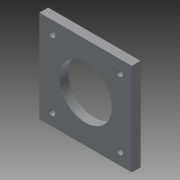
# Autodesk Inventor part: ZMotorMount
Saved by Autodesk Inventor 2015 (Build 190159000, 159)
## iProperties
Created: 2014-08-12
Part Number: ZMotorMount
Material: Generic
Document SubType Name: Modeling
Designer: Jack
Density: 1 g/cm^3
Appearance: Default
Author: Jack
Autodesk Inventor part; units mm, degrees
ref_plane "YZ Plane" through (0, 0, 0) normal (1, 0, 0) x (0, 1, 0)
ref_plane "XZ Plane" through (0, 0, 0) normal (0, 1, 0) x (-1, 0, 0)
ref_plane "XY Plane" through (0, 0, 0) normal (0, 0, 1) x (1, 0, 0)
sketch "Sketch1" plane through (0, 0, 0) normal (0, 1, 0) x (-1, 0, 0)
  line L0 (0, 0) -> (42.3, 0)
  line L1 (42.3, 0) -> (42.3, -42.3)
  line L2 (42.3, -42.3) -> (0, -42.3)
  line L3 (0, -42.3) -> (0, 0)
  dimension "d0" = 42.3
  constraints: 8 end point, 2 parallel, 2 perpendicular, 1 horizontal
  measures "d0" distance of L0.start L0.end
extrude "Extrusion1" add sketch "Sketch1" along normal blind 4
sketch "Sketch2" plane through (0, 4, 0) normal (0, 1, 0) x (1, 0, 0)
  line L0 (0, 42.3) -> (-42.3, 42.3) projected
  line L1 (-42.3, 42.3) -> (-42.3, 0) projected
  circle A0 centre (-36.65, 5.65) radius 1.5
  circle A1 centre (-5.65, 5.65) radius 1.5
  circle A2 centre (-36.65, 36.65) radius 1.5
  circle A3 centre (-5.65, 36.65) radius 1.5
  dimension "d3" = 3
  dimension "d5" = 31
  dimension "d6" = 31
  dimension "d7" = 5.65
  dimension "d8" = 5.65
  constraints: 4 centre point, 3 equal radius, 2 horizontal alignment, 2 vertical alignment
  measures "d3" diameter of A0
  measures "d5" distance of A0.centre A1.centre
  measures "d6" distance of A2.centre A0.centre
  measures "d7" distance from line of L0 A2.centre
  measures "d8" distance from line of L1 A0.centre
extrude "Extrusion2" cut sketch "Sketch2" against normal up to next
sketch "Sketch3" plane through (0, 4, 0) normal (0, 1, 0) x (1, 0, 0)
  line L0 (-42.3, 0) -> (0, 0) projected
  line L1 (-42.3, 42.3) -> (-42.3, 0) projected
  circle A0 centre (-21.15, 21.15) radius 12
  dimension "d11" = 24
  dimension "d12" = 21.15
  dimension "d13" = 21.15
  constraints: 1 centre point
  measures "d11" diameter of A0
  measures "d12" distance from line of L0 A0.centre
  measures "d13" distance from line of L1 A0.centre
extrude "Extrusion3" cut sketch "Sketch3" against normal up to next
body "Solid1"
